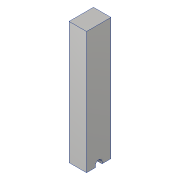
# Autodesk Inventor part: 10-002-ARM
Saved by Autodesk Inventor 2018 (Build 220112000, 112)
## iProperties
Created: 2017-07-19
Part Number: 10-002-ARM
Material: Aluminum 6061
Document SubType Name: Modeling
Designer: feesmrt
Density: 2.7 g/cm^3
Appearance: Aluminum - Flat
Author: feesmrt
Autodesk Inventor part; units mm, degrees
ref_plane "YZ Plane" through (0, 0, 0) normal (1, 0, 0) x (0, 1, 0)
ref_plane "XZ Plane" through (0, 0, 0) normal (0, 1, 0) x (-1, 0, 0)
ref_plane "XY Plane" through (0, 0, 0) normal (0, 0, 1) x (1, 0, 0)
sketch "Sketch1" plane through (0, 0, 0) normal (0, 0, 1) x (1, 0, 0)
  line L0 (-30.1, 0) -> (30.1, 0) construction
  line L1 (0, 42) -> (0, -42) construction
  line L2 (-21.5, -30) -> (21.5, -30)
  line L3 (21.5, -30) -> (21.5, 30)
  line L4 (21.5, 30) -> (-21.5, 30)
  line L5 (-21.5, 30) -> (-21.5, -30)
  line L6 (-21.5, -30) -> (21.5, 30) construction
  line L7 (21.5, -30) -> (-21.5, 30) construction
  point P0 (0, 0)
  dimension "d0" = 43
  dimension "d1" = 60
  constraints: 12 end point, 2 midpoint, 2 parallel, 1 horizontal, 1 perpendicular
  measures "d0" distance of L3.end L4.end
  measures "d1" distance of L2.end L3.end
extrude "Extrusion1" add sketch "Sketch1" along normal blind 300
sketch "Sketch4" plane through (-21.5, -30, 0) normal (-1, 0, 0) x (0, 0, 1)
  line L0 (0, 60) -> (0, 0) construction
  line L1 (-60, 30) -> (360, 30) construction
  line L2 (0, 38) -> (5, 38)
  line L3 (13, 30) -> (13, 30)
  line L4 (5, 22) -> (0, 22)
  line L5 (0, 22) -> (0, 38)
  arc A0 (13, 30) -> (5, 38) centre (5, 30) ccw
  arc A1 (5, 22) -> (13, 30) centre (5, 30) ccw
  point P0 (0, 30)
  point P1 (13, 22)
  point P2 (13, 38)
  dimension "d7" = 16
  dimension "d8" = 13
  dimension "d9" = 8
  constraints: 8 end point, 5 point on line, 4 point on circle, 4 tangent, 2 centre point, 2 parallel, 1 concentric, 1 horizontal, 1 perpendicular, 1 other
  measures "d7" distance of point (13, 38) point (13, 22)
  measures "d8" distance of L2.start point (13, 38)
  measures "d9" radius of A0
extrude "Extrusion3" cut sketch "Sketch4" against normal through all
sketch "Sketch5" plane through (0, 0, 0) normal (0, 0, -1) x (-1, 0, 0)
  line L0 (0, -42) -> (0, 42) construction
  line L1 (-30.1, 0) -> (30.1, 0) construction
  line L2 (-10.75, -19) -> (10.75, -19) construction
  line L3 (10.75, -19) -> (10.75, 19) construction
  line L4 (10.75, 19) -> (-10.75, 19) construction
  line L5 (-10.75, 19) -> (-10.75, -19) construction
  line L6 (-10.75, -19) -> (10.75, 19) construction
  line L7 (10.75, -19) -> (-10.75, 19) construction
  line L8 (21.5, -30) -> (-21.5, -30) projected
  line L9 (-21.5, 30) -> (21.5, 30) projected
  line L10 (21.5, -8) -> (-21.5, -8) construction
  line L11 (-21.5, 8) -> (21.5, 8) construction
  point P0 (0, 0)
  dimension "d12" = 21.5
  dimension "d13" = 38
  dimension "d14" = 60
  dimension "d15" = 16
  dimension "d16" = 43
  constraints: 12 end point, 4 coincident, 2 midpoint, 2 parallel, 1 horizontal, 1 perpendicular
  measures "d12" distance of L3.end L4.end
  measures "d13" distance of L2.end L3.end
  measures "d14" distance between parallel lines of L8 L9
  measures "d15" distance between parallel lines of L10 L11
  measures "d16" distance of L8.start L8.end
hole "Hole1" at (10.75, 19, 0) at (-10.75, 19, 0) at (-10.75, -19, 0) at (10.75, -19, 0) direction (0, 0, 1) diameter 4.134 depth 14.2 tip angle 118 countersink diameter 5 countersink angle 90 thread size "M5x0.8" class "6H" standard "ISO Metric profile"
equation "\"d9\" = 0.5 * d7"
equation "\"d12\" = 0.5 * d16"
equation "\"d13\" = 0.5 * d14 + 0.5 * d15"
body "Solid1"
